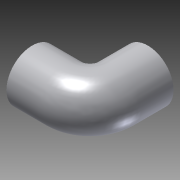
# Autodesk Inventor part: 0.5 Elbow
Saved by Autodesk Inventor 2013 (Build 170138000, 138)
## iProperties
Created: 2014-08-06
Part Number: 0.5 Elbow
Material: PVC-Piping
Document SubType Name: Modeling
Designer: Kyle
Density: 1 g/cm^3
Author: Kyle
Autodesk Inventor part; units mm, degrees
ref_plane "YZ Plane" through (0, 0, 0) normal (1, 0, 0) x (0, 1, 0)
ref_plane "XZ Plane" through (0, 0, 0) normal (0, 1, 0) x (-1, 0, 0)
ref_plane "XY Plane" through (0, 0, 0) normal (0, 0, 1) x (1, 0, 0)
sketch "Sketch1" plane through (0, 0, 0) normal (0, 0, 1) x (1, 0, 0)
  circle A0 centre (-3.105, 0) radius 13.97
  circle A1 centre (-3.105, 0) radius 10.414
  point P0 (0, 0)
  dimension "d0" = 27.94
  dimension "d2" = 20.828
  constraints: 2 centre point
  measures "d0" diameter of A0
  measures "d2" diameter of A1
extrude "Extrusion1" add sketch "Sketch1" along normal blind 17.526
sketch "Sketch2" plane through (-3.105, 0, 17.526) normal (0, 0, 1) x (1, 0, 0)
  circle A0 centre (0, 0) radius 10.414 projected
  circle A1 centre (0, 0) radius 13.97 projected
  line L0 (-13.97, 13.97) -> (-13.97, -13.97)
  line L1 (-13.97, -13.97) -> (13.97, -13.97)
  point P0 (3.105, 0)
  constraints: 4 end point, 1 perpendicular, 1 vertical
revolve "Revolution1" add sketch "Sketch2" angle 90 about axis through (-17.075, 13.97, 17.526) along (0, -1, 0) contours A1
sketch "Sketch3" plane through (-17.075, 0, 31.496) normal (-1, 0, 0) x (0, 0, 1)
  circle A0 centre (0, 0) radius 10.414 projected
  circle A1 centre (0, 0) radius 13.97 projected
  point P0 (-13.97, 0)
  point P1 (-31.496, 0)
  constraints: 1 horizontal alignment
extrude "Extrusion2" add sketch "Sketch3" along normal blind 17.526
sketch "Sketch4" plane through (-34.601, 0, 31.496) normal (-1, 0, 0) x (0, 0, 1)
  circle A0 centre (0, 0) radius 10.414 projected
  circle A1 centre (0, 0) radius 13.97 projected
  circle A2 centre (0, 0) radius 10.795
  point P0 (-31.496, 0)
  dimension "d8" = 21.59
  constraints: 1 centre point, 1 coincident
  measures "d8" diameter of A2
extrude "Extrusion3" cut sketch "Sketch4" against normal blind 19.05 contours A2
sketch "Sketch5" plane through (-3.105, 0, 0) normal (0, 0, -1) x (-1, 0, 0)
  circle A0 centre (0, 0) radius 10.414 projected
  circle A1 centre (0, 0) radius 13.97 projected
  circle A2 centre (0, 0) radius 10.795
  point P0 (-3.105, 0)
  dimension "d12" = 21.59
  constraints: 1 centre point, 1 coincident
  measures "d12" diameter of A2
extrude "Extrusion4" cut sketch "Sketch5" against normal blind 19.05 contours A2
body "Solid1"
